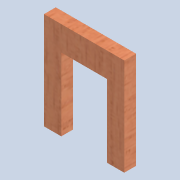
# Autodesk Inventor part: 0005-10-026 Suport DC in
Saved by Autodesk Inventor 2020 (Build 240168000, 168)
## iProperties
Created: 2020-12-18
Part Number: 0005-10-026 Suport DC in
Material: Wood (Cherry)
Document SubType Name: Modeling
Designer: Iulian Bors
Density: 0.63 g/cm^3
Appearance: White Oak - Natural Medium Gloss
Mass: 10.4266 g
Surface Area: 68.5355 cm^2
Volume: 16.5502 cm^3
Author: Iulian Bors
Subject: 026
Autodesk Inventor part; units mm, degrees
ref_plane "YZ Plane" through (0, 0, 0) normal (1, 0, 0) x (0, 1, 0)
ref_plane "XZ Plane" through (0, 0, 0) normal (0, 1, 0) x (-1, 0, 0)
ref_plane "XY Plane" through (0, 0, 0) normal (0, 0, 1) x (1, 0, 0)
sketch "Sketch1" plane through (0, 0, 0) normal (0, 0, 1) x (1, 0, 0)
  line L0 (-27.25, 33) -> (27.25, 33)
  line L1 (27.25, 33) -> (27.25, -33)
  line L2 (27.25, -33) -> (-27.25, -33)
  line L3 (-27.25, -33) -> (-27.25, 33)
  point P0 (0, 0)
  point P1 (0, 33)
  point P2 (-27.25, 0)
  dimension "d0" = 54.5
  dimension "d1" = 66
  constraints: 8 end point, 2 midpoint, 2 parallel, 1 horizontal, 1 horizontal alignment, 1 perpendicular, 1 vertical alignment
  measures "d0" distance of L0.start L0.end
  measures "d1" distance of L2.end L0.start
extrude "Extrusion1" add sketch "Sketch1" along normal blind 8
sketch "Sketch2" plane through (0, 0, 8) normal (0, 0, 1) x (1, 0, 0)
  line L0 (27.25, 33) -> (-27.25, 33) projected
  line L1 (-27.25, 33) -> (-27.25, -33) projected
  line L2 (-7.6866, 14.25) -> (7.6866, 14.25) projected
  line L3 (-12.41, -5.57) -> (-12.41, -14.27) projected
  line L4 (-13.515, -31) -> (-13.515, 8.4216) projected
  line L5 (13.515, 8.4216) -> (13.515, -31) projected
  line L6 (-27.25, -33) -> (27.25, -33) projected
  line L7 (-15.515, 16.25) -> (15.515, 16.25)
  line L8 (15.515, 16.25) -> (15.515, -33)
  line L9 (15.515, -33) -> (-15.515, -33)
  line L10 (-15.515, -33) -> (-15.515, 16.25)
  line L11 (-27.25, -33) -> (27.25, -33) projected
  point P0 (-27.25, 0)
  dimension "d29" = 2
  dimension "d30" = 2
  dimension "d32" = 2
  constraints: 8 end point, 2 parallel, 1 collinear, 1 horizontal, 1 midpoint, 1 perpendicular
  measures "d29" distance between parallel lines of L2 L7
  measures "d30" distance between parallel lines of L4 L10
  measures "d32" distance between parallel lines of L8 L5
extrude "Extrusion2" cut sketch "Sketch2" against normal through all
equation "\"d32\" = d30"
body "Solid1"
